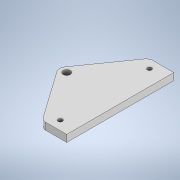
# Autodesk Inventor part: Tapa
Saved by Autodesk Inventor 2020.3 (Build 243373000, 373)
## iProperties
Created: 2020-07-26
Part Number: Tapa
Material: Generic
Document SubType Name: Modeling
Designer: juanp
Density: 1 g/cm^3
Appearance: Default
Author: juanp
Autodesk Inventor part; units mm, degrees
ref_plane "YZ Plane" through (0, 0, 0) normal (1, 0, 0) x (0, 1, 0)
ref_plane "XZ Plane" through (0, 0, 0) normal (0, 1, 0) x (-1, 0, 0)
ref_plane "XY Plane" through (0, 0, 0) normal (0, 0, 1) x (1, 0, 0)
sketch "Sketch1" plane through (0, 0, 0) normal (0, 1, 0) x (-1, 0, 0)
  circle A0 centre (0, 0) radius 30.16 construction
  circle A1 centre (0, 0) radius 38.16 construction
  line L0 (38.16, 38.16) -> (0, 38.16) construction
  line L1 (-38.16, 38.16) -> (-38.16, -38.16)
  line L2 (-38.16, -38.16) -> (0, -38.16)
  line L3 (38.16, -38.16) -> (38.16, 38.16) construction
  line L4 (38.16, 38.16) -> (-38.16, -38.16) construction
  line L5 (-38.16, 38.16) -> (38.16, -38.16) construction
  circle A2 centre (0, 0) radius 2.55
  line L6 (-49.3749, 20.3741) -> (-55.9459, 20.3741) construction
  circle A3 centre (-27.211, 31.78) radius 1.55
  line L7 (0, 38.16) -> (-38.16, 38.16)
  line L8 (0, -38.16) -> (38.16, -38.16) construction
  line L9 (-38.16, 0) -> (-46.6807, 0) construction
  circle A4 centre (-27.211, -31.78) radius 1.55
  arc A5 (0, -5) -> (-3.5355, -3.5355) centre (0, 0) ccw
  arc A6 (-3.5355, -3.5355) -> (0, -5) centre (0, 0) ccw
  line L10 (-27.211, 31.78) -> (-16.262, 31.78) construction
  line L11 (-16.262, 38.16) -> (-16.262, 0) construction
  line L12 (-16.262, 31.78) -> (4.0882, 2.8786)
  line L13 (-16.262, 31.78) -> (-20.7543, 38.16)
  line L14 (-16.262, -31.78) -> (4.0882, -2.8786)
  line L15 (-16.262, -31.78) -> (-20.7543, -38.16)
  point P0 (-20.7543, -38.16)
  point P1 (4.0882, -2.8786)
  dimension "d0" = 60.32
  dimension "d1" = 8
  dimension "d2" = 5.1
  dimension "d3" = 6.38
  dimension "d4" = 10.949
  dimension "d5" = 3.1
  dimension "d6" = 10
  dimension "d10" = 10.949
  constraints: 32 end point, 7 centre point, 7 point on circle, 5 coincident, 5 horizontal, 5 parallel, 4 point on line, 4 symmetric about line, 4 tangent, 3 midpoint, 2 perpendicular, 1 collinear, 1 vertical, 1 other
  measures "d0" diameter of A0
  measures "d1" radial gap between concentric circles of A0 A1
  measures "d2" diameter of A2
  measures "d3" distance from line of L0 point (-27.211, 31.78)
  measures "d4" distance from line of L1 point (-27.211, 31.78)
  measures "d5" diameter of A3
  measures "d6" diameter of A5
  measures "d10" distance of L10.start L10.end
extrude "Extrusion1" add sketch "Sketch1" along normal blind 5
fillet "Fillet1" radius 5 2 edges at (20.7543, 2.5, 38.16) (20.7543, 2.5, -38.16)
body "Solid1"
